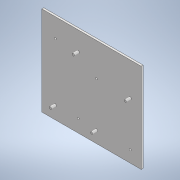
# Autodesk Inventor part: Electrical Box
Saved by Autodesk Inventor 2020.2 (Build 242310000, 310)
## iProperties
Created: 2020-04-13
Part Number: Electrical Box
Material: Generic
Document SubType Name: Modeling
Designer: Josiah
Density: 1 g/cm^3
Appearance: Default
Author: Josiah
Autodesk Inventor part; units mm, degrees
ref_plane "YZ Plane" through (0, 0, 0) normal (1, 0, 0) x (0, 1, 0)
ref_plane "XZ Plane" through (0, 0, 0) normal (0, 1, 0) x (-1, 0, 0)
ref_plane "XY Plane" through (0, 0, 0) normal (0, 0, 1) x (1, 0, 0)
sketch "Sketch1" plane through (0, 0, 0) normal (0, 0, 1) x (1, 0, 0)
  line L0 (-50, 45) -> (50, 45)
  line L1 (50, 45) -> (50, -45)
  line L2 (50, -45) -> (-50, -45)
  line L3 (-50, -45) -> (-50, 45)
  line L4 (-50, -45) -> (50, 45) construction
  point P0 (0, 0)
  point P1 (0, 0)
  dimension "d0" = 100
  dimension "d1" = 90
  constraints: 10 end point, 2 parallel, 1 coincident, 1 horizontal, 1 midpoint, 1 perpendicular, 1 other
  measures "d0" distance of L0.start L0.end
  measures "d1" distance of L0.end L1.end
extrude "Extrusion1" add sketch "Sketch1" along normal blind 2
sketch "Sketch2" plane through (0, 0, 2) normal (0, 0, 1) x (1, 0, 0)
  circle A0 centre (39.0346, -33.2431) radius 1.25 projected
  circle A1 centre (5.1346, -33.2431) radius 1.25 projected
  circle A2 centre (5.1346, 11.6569) radius 1.25 projected
  circle A3 centre (39.0346, 11.6569) radius 1.25 projected
  circle A4 centre (-13.3759, -32.147) radius 1.325 projected
  circle A5 centre (-36.4259, -32.147) radius 1.325 projected
  circle A6 centre (-13.3759, 25.903) radius 1.325 projected
  circle A7 centre (-36.4259, 25.903) radius 1.325 projected
  circle A8 centre (39.0346, -33.2431) radius 1
  circle A9 centre (5.1346, -33.2431) radius 1
  circle A10 centre (-13.3759, -32.147) radius 1
  circle A11 centre (-36.4259, -32.147) radius 1
  circle A12 centre (-13.3759, 25.903) radius 1
  circle A13 centre (-36.4259, 25.903) radius 1
  circle A14 centre (5.1346, 11.6569) radius 1
  circle A15 centre (39.0346, 11.6569) radius 1
  point P0 (0, 0)
  dimension "d4" = 2
  dimension "d5" = 2
  dimension "d6" = 2
  dimension "d7" = 2
  dimension "d8" = 2
  dimension "d9" = 2
  dimension "d10" = 2
  dimension "d11" = 2
  constraints: 8 centre point, 8 coincident
  measures "d4" diameter of A8
  measures "d5" diameter of A9
  measures "d6" diameter of A10
  measures "d7" diameter of A11
  measures "d8" diameter of A12
  measures "d9" diameter of A13
  measures "d10" diameter of A14
  measures "d11" diameter of A15
extrude "Extrusion2" cut sketch "Sketch2" against normal blind 10 contours A8 | A10 | A13 | A14
sketch "Sketch3" plane through (0, 0, 2) normal (0, 0, 1) x (1, 0, 0)
  circle A0 centre (39.0346, 11.6569) radius 1.25 projected
  circle A1 centre (5.1346, -33.2431) radius 1.25 projected
  circle A2 centre (-36.4259, -32.147) radius 1.325 projected
  circle A3 centre (-13.3759, 25.903) radius 1.325 projected
  circle A4 centre (5.1346, -33.2431) radius 1.1
  circle A5 centre (-36.4259, -32.147) radius 1.175
  circle A6 centre (-13.3759, 25.903) radius 1.175
  circle A7 centre (39.0346, 11.6569) radius 1.1
  point P0 (0, 0)
  dimension "d14" = 0.15
  dimension "d15" = 0.15
  dimension "d16" = 0.15
  dimension "d17" = 0.15
  constraints: 4 centre point
  measures "d14" radial gap between concentric circles of A1 A4
  measures "d15" radial gap between concentric circles of A2 A5
  measures "d16" radial gap between concentric circles of A3 A6
  measures "d17" radial gap between concentric circles of A0 A7
extrude "Extrusion3" add sketch "Sketch3" along normal blind 5 contours A4 | A5 | A6 | A7
equation "\"d15\" = d14"
equation "\"d16\" = d14"
equation "\"d17\" = d14"
body "Solid1"
